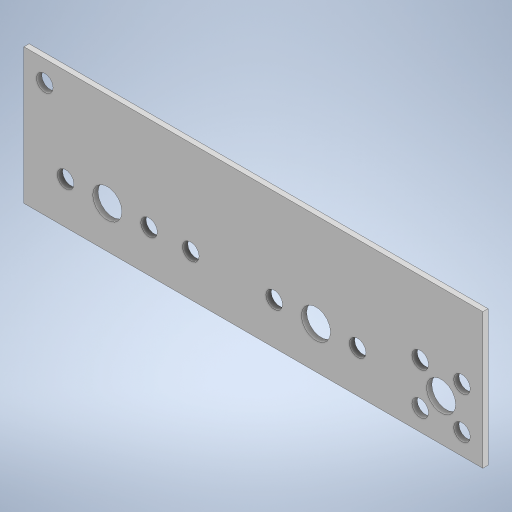
# Autodesk Inventor part: flatPoly1ForCNC
Saved by Autodesk Inventor 2023.4 (Build 274418000, 418)
## iProperties
Created: 2023-12-19
Part Number: flatPoly1ForCNC
Material: Generic
Document SubType Name: Modeling
Designer: Meer
Density: 1 g/cm^3
Appearance: Default
Author: Meer
Autodesk Inventor part; units mm, degrees
ref_plane "YZ Plane" through (0, 0, 0) normal (1, 0, 0) x (0, 1, 0)
ref_plane "XZ Plane" through (0, 0, 0) normal (0, 1, 0) x (-1, 0, 0)
ref_plane "XY Plane" through (0, 0, 0) normal (0, 0, 1) x (1, 0, 0)
sketch "Sketch1" plane through (0, 0, 0) normal (0, 0, 1) x (1, 0, 0)
  line L0 (0, 0) -> (139.7, 0)
  line L1 (139.7, 0) -> (139.7, 41.275)
  line L2 (139.7, 41.275) -> (0, 41.275)
  line L3 (0, 41.275) -> (0, 0)
  circle A0 centre (12.7, 12.7) radius 2.54
  circle A1 centre (25.4, 12.7) radius 4.445
  circle A2 centre (38.1, 12.7) radius 2.54
  circle A3 centre (50.8, 12.7) radius 2.54
  circle A4 centre (76.2, 12.7) radius 2.54
  circle A5 centre (88.9, 12.7) radius 4.445
  circle A6 centre (101.6, 12.7) radius 2.54
  circle A7 centre (127, 12.7) radius 4.445
  circle A8 centre (133.35, 19.05) radius 2.54
  circle A9 centre (133.35, 6.35) radius 2.54
  circle A10 centre (120.65, 6.35) radius 2.54
  circle A11 centre (120.65, 19.05) radius 2.54
  circle A12 centre (6.35, 34.925) radius 2.54
  dimension "d0" = 139.7
  dimension "d1" = 41.275
  dimension "d6" = 5.08
  dimension "d12" = 8.89
  dimension "d13" = 5.08
  dimension "d14" = 5.08
  dimension "d15" = 5.08
  dimension "d19" = 8.89
  dimension "d20" = 5.08
  dimension "d21" = 8.89
  dimension "d24" = 5.08
  dimension "d28" = 5.08
  dimension "d29" = 5.08
  dimension "d30" = 5.08
  dimension "d34" = 5.08
  constraints: 13 centre point, 8 end point, 2 parallel, 1 horizontal, 1 perpendicular
  measures "d0" distance of L2.end L1.end
  measures "d1" distance of L0.end L1.end
  measures "d6" diameter of A0
  measures "d12" diameter of A1
  measures "d13" diameter of A2
  measures "d14" diameter of A3
  measures "d15" diameter of A4
  measures "d19" diameter of A5
  measures "d20" diameter of A6
  measures "d21" diameter of A7
  measures "d24" diameter of A8
  measures "d28" diameter of A9
  measures "d29" diameter of A10
  measures "d30" diameter of A11
  measures "d34" diameter of A12
extrude "Extrusion1" add sketch "Sketch1" along normal blind 1.5875
body "Solid1"
